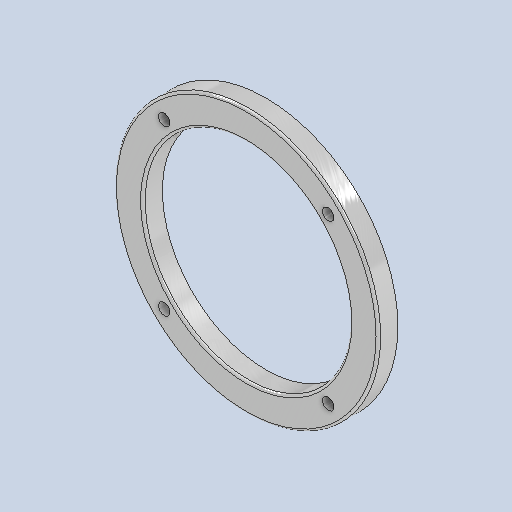
# Autodesk Inventor part: turntable_in_8_23
Saved by Autodesk Inventor 2022 (Build 260153070, 153G)
## iProperties
Created: 2021-08-23
Part Number: turntable_in_8_23
Material: アルミニウム 6061-AHC
Document SubType Name: Modeling
Designer: sky
Density: 2.7 g/cm^3
Appearance: 機械加工 - アルミニウム
Mass: 90.2019 g
Surface Area: 136.251 cm^2
Volume: 33.4081 cm^3
Author: sky
Autodesk Inventor part; units mm, degrees
ref_plane "YZ Plane" through (0, 0, 0) normal (1, 0, 0) x (0, 1, 0)
ref_plane "XZ Plane" through (0, 0, 0) normal (0, 1, 0) x (-1, 0, 0)
ref_plane "XY Plane" through (0, 0, 0) normal (0, 0, 1) x (1, 0, 0)
sketch "スケッチ1" plane through (0, 0, 0) normal (0, 0, 1) x (1, 0, 0)
  circle A0 centre (0, 0) radius 45
  circle A1 centre (0, 0) radius 57.5
  dimension "d0" = 90
  dimension "d1" = 115
  constraints: 2 centre point, 2 coincident
  measures "d0" diameter of A0
  measures "d1" diameter of A1
extrude "押し出し1" add sketch "スケッチ1" along normal blind 8.5
sketch "スケッチ2" plane through (0, 0, 8.5) normal (0, 0, 1) x (1, 0, 0)
  line L0 (0, 0) -> (35.7, 0)
  line L1 (35.7, 0) -> (35.7, -35.7)
  line L2 (35.7, -35.7) -> (0, -35.7)
  line L3 (0, -35.7) -> (0, 0)
  point P0 (35.7, 35.7)
  point P1 (-35.7, 35.7)
  point P2 (-35.7, -35.7)
  dimension "d13" = 35.7
  dimension "d14" = 35.7
  dimension "d17" = 360
  constraints: 8 end point, 2 coincident, 2 parallel, 1 horizontal, 1 perpendicular, 5 other
  measures "d13" distance of L1.end L2.end
  measures "d14" distance of L0.end L1.end
hole "穴1" at (-35.7, 35.7, 8.5) at (35.7, 35.7, 8.5) at (-35.7, -35.7, 8.5) at (35.7, -35.7, 8.5) direction (0, 0, -1) diameter 5 end through all
fillet "フィレット1" radius 1 2 edges at (-45, 0, 8.5) (-57.5, 0, 8.5)
